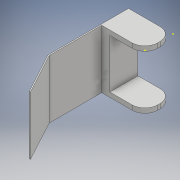
# Autodesk Inventor part: CRANEHAND
Saved by Autodesk Inventor 2017 (Build 210142000, 142)
## iProperties
Part Number: CRANEHAND
Material: 一般
Document SubType Name: Modeling
Designer: rsdlab
Density: 1 g/cm^3
Appearance: 既定
Author: rsdlab
Autodesk Inventor part; units mm, degrees
ref_plane "YZ Plane" through (0, 0, 0) normal (1, 0, 0) x (0, 1, 0)
ref_plane "XZ Plane" through (0, 0, 0) normal (0, 1, 0) x (-1, 0, 0)
ref_plane "XY Plane" through (0, 0, 0) normal (0, 0, 1) x (1, 0, 0)
sketch "スケッチ1" plane through (0, 0, 0) normal (0, 1, 0) x (-1, 0, 0)
  line L0 (0, 0) -> (0.37, 0)
  line L1 (0.37, 0) -> (0.37, -0.04)
  line L2 (0.37, -0.04) -> (0, -0.04)
  line L3 (0, -0.04) -> (0, 0)
  line L4 (0.37, -0.04) -> (0.3, -0.04)
  line L5 (0.3, -0.04) -> (0.3, -0.46)
  line L6 (0.3, -0.46) -> (0.37, -0.46)
  line L7 (0.37, -0.46) -> (0.37, -0.04)
  line L8 (0.37, -0.46) -> (0, -0.46)
  line L9 (0, -0.46) -> (0, -0.5)
  line L10 (0, -0.5) -> (0.37, -0.5)
  line L11 (0.37, -0.5) -> (0.37, -0.46)
  dimension "d2" = 0.37
  dimension "d3" = 0.04
  dimension "d4" = 0.07
  dimension "d5" = 0.42
  dimension "d6" = 0.04
  constraints: 24 end point, 6 parallel, 3 horizontal, 3 perpendicular
  measures "d2" distance of L1.end L2.end
  measures "d3" distance of L0.end L1.end
  measures "d4" distance of L6.end L5.end
  measures "d5" distance of L5.end L4.end
  measures "d6" distance of L9.end L8.end
extrude "押し出し1" add sketch "スケッチ1" against normal blind 0.24
sketch "スケッチ2" plane through (0, -0.24, 0) normal (0, -1, 0) x (1, 0, 0)
  point P0 (0, 0)
sketch "スケッチ3" plane through (0, -0.24, 0) normal (0, -1, 0) x (1, 0, 0)
  point P0 (0, 0)
sketch "スケッチ4" plane through (0, -0.24, 0) normal (0, -1, 0) x (1, 0, 0)
  point P0 (0, 0)
fillet "フィレット1" radius 0.11 4 edges at (0, -0.24, -0.48) (0, 0, -0.48) (0, -0.24, -0.02) (0, 0, -0.02)
sketch "スケッチ5" plane through (-0.37, 0, -0.5) normal (-1, 0, 0) x (0, 0, 1)
  line L0 (0.5, 0) -> (0.5, -0.24) projected
  line L1 (0, 0) -> (0, -0.24) projected
  line L2 (0.5, 0) -> (0, 0)
  line L3 (0, 0) -> (0, -0.24)
  line L4 (0, -0.24) -> (0.5, -0.24)
  line L5 (0.5, -0.24) -> (0.5, 0)
  constraints: 8 end point, 2 parallel, 1 horizontal, 1 perpendicular
extrude "押し出し2" add sketch "スケッチ5" along normal blind 0.01
sketch "スケッチ6" plane through (0, -0.24, 0) normal (0, -1, 0) x (1, 0, 0)
  line L0 (-0.38, -0.5) -> (-0.38, 0) projected
  line L1 (-0.11, -0.5) -> (-0.38, -0.5) projected
  line L2 (-0.38, 0) -> (-0.37, 0)
  line L3 (-0.37, 0) -> (-0.37, -0.5)
  line L4 (-0.37, -0.5) -> (-0.38, -0.5)
  line L5 (-0.38, -0.5) -> (-0.38, 0)
  point P0 (0, 0)
  dimension "d12" = 0.01
  constraints: 8 end point, 2 parallel, 1 horizontal, 1 perpendicular, 1 point on line
  measures "d12" distance of L3.end L4.end
extrude "押し出し3" add sketch "スケッチ6" along normal blind 0.45
sketch "スケッチ7" plane through (0, -0.69, 0) normal (0, -1, 0) x (1, 0, 0)
  line L0 (-0.38, 0) -> (-0.38, -0.5) projected
  line L1 (-0.11, -0.5) -> (-0.38, -0.5) projected
  line L2 (-0.38, 0) -> (-0.18, 0)
  line L3 (-0.18, 0) -> (-0.18, -0.5)
  line L4 (-0.18, -0.5) -> (-0.38, -0.5)
  line L5 (-0.38, -0.5) -> (-0.38, 0)
  point P0 (0, 0)
  dimension "d15" = 0.2
  constraints: 8 end point, 2 parallel, 1 horizontal, 1 perpendicular, 1 point on line
  measures "d15" distance of L3.end L4.end
extrude "押し出し4" add sketch "スケッチ7" along normal blind 0.35
sketch "スケッチ8" plane through (-0.38, 0, 0) normal (0, 0, 1) x (1, 0, 0)
  point P0 (0.38, 0)
sketch "スケッチ9" plane through (-0.38, 0, 0) normal (0, 0, 1) x (1, 0, 0)
  point P0 (0.38, 0)
sketch "スケッチ10" plane through (-0.38, 0, 0) normal (0, 0, 1) x (1, 0, 0)
  point P0 (0.38, 0)
chamfer "面取り1" distance 0.19 distance2 0.35 1 edges at (-0.38, -1.04, -0.25) measured on face at (-0.2467, -1.04, -0.3333)
chamfer "面取り2" distance 0.35 distance2 0.19 1 edges at (-0.18, -0.69, -0.25) measured on face at (-0.18, -0.8067, -0.3333)
